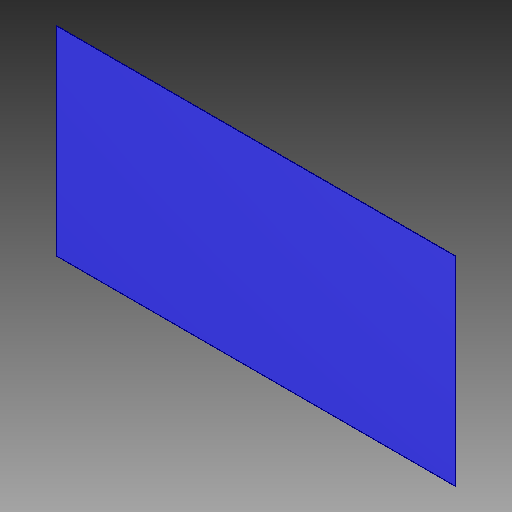
# Autodesk Inventor part: 16_000
Saved by Autodesk Inventor 2017 (Build 210142000, 142)
## iProperties
Created: 2019-06-13
Part Number: 16_000
Material: Generic
Document SubType Name: Modeling
Designer: Marc
Density: 1 g/cm^3
Appearance: HC49U-V, 16_000
Author: Marc
Autodesk Inventor part; units mm, degrees
ref_plane "YZ Plane" through (0, 0, 0) normal (1, 0, 0) x (0, 1, 0)
ref_plane "XZ Plane" through (0, 0, 0) normal (0, 1, 0) x (-1, 0, 0)
ref_plane "XY Plane" through (0, 0, 0) normal (0, 0, 1) x (1, 0, 0)
sketch "HC49U-V, 16_000_66" plane through (0, 0, 0) normal (0, 0, 1) x (1, 0, 0)
  line L0 (-5.588, 2.794) -> (5.588, 2.794)
  line L1 (5.588, 2.794) -> (5.588, -2.794)
  line L2 (5.588, -2.794) -> (-5.588, -2.794)
  line L3 (-5.588, -2.794) -> (-5.588, 2.794)
  constraints: 8 end point
extrude "Extrusion1" add sketch "HC49U-V, 16_000_66" along normal blind 0.01
body "Solid1"
